timer_indicator_disk_v2 (Autodesk Fusion 360 design; units mm, degrees)
Autodesk Fusion 360 part; units mm, degrees
note: some values were not read from the file. Chosen so that the rebuilt part matches the saved one: that a step has no effect.
sketch "Sketch1" plane through (0, 0, 0) normal (0, 0, 1) x (1, 0, 0)
  circle A0 centre (0, 0) radius 65
  line L0 (2.125, -0.975) -> (2.125, 0.975)
  arc A1 (2.125, 0.975) -> (-2.125, 0.975) centre (0, 0.975) ccw
  line L1 (-2.125, 0.975) -> (-2.125, -0.975)
  arc A2 (-2.125, -0.975) -> (2.125, -0.975) centre (0, -0.975) ccw
  line L2 (0, -0.975) -> (0, 0.975) construction
  line L3 (0, 3.1) -> (0, -3.1) construction
  line L4 (0, 0) -> (65, 0) construction
  line L5 (0, 0) -> (-65, 0) construction
  circle A3 centre (-7.25, 0) radius 1.125
  circle A4 centre (7.25, 0) radius 1.125
  line L6 (-6.125, 0) -> (-2.125, 0) construction
  line L7 (6.125, 0) -> (2.125, 0) construction
  line L8 (12.5, 0) -> (5, -11.8216)
  arc A5 (12.5, 0) -> (-12.5, 0) centre (0, 0) ccw
  line L9 (5, -11.8216) -> (-5, -11.8216)
  line L10 (0, -0.975) -> (0, -65) construction
  line L11 (0, -35.0581) -> (0, -65) construction
  line L12 (-12.5, 0) -> (-5, -11.8216)
  arc A6 (16.4537, -1.2347) -> (-16.5, 0) centre (0, 0) ccw
  line L13 (16.4537, -1.2347) -> (9.6102, -12.0216)
  line L14 (9.6102, -12.0216) -> (-0.3898, -12.0216)
  arc A7 (-0.3898, -12.0216) -> (-0.3898, -21.6037) centre (-0.3898, -16.8127) ccw
  line L15 (-0.3898, -21.6037) -> (0.0565, -21.6037)
  line L16 (0.0565, -21.6037) -> (0.0565, -65)
  line L17 (5, -11.8216) -> (-0.3898, -11.8216)
  arc A8 (-0.3898, -11.8216) -> (-0.1435, -21.7976) centre (-0.3898, -16.8127) ccw
  line L18 (-0.1435, -21.7976) -> (-0.1435, -64.9998)
  line L19 (0.0565, -65) -> (-0.0002, -73)
  arc A9 (-0.0002, -73) -> (3.9997, -73.0283) centre (1.9998, -73.0141) ccw
  line L20 (3.9997, -73.0283) -> (4.0575, -64.8732)
  arc A10 (-16.5, 0) -> (-12.5, 0) centre (-14.5, 0) ccw
  line L21 (0, 12.5) -> (39.231, 12.5) construction
  line L22 (0, -11.8216) -> (39.4618, -11.8216) construction
  dimension "d1" = 130
  dimension "d2" = 4.25
  dimension "d4" = 6.2
  dimension "d5" = 2.25
  dimension "d6" = 2.25
  dimension "d7" = 4
  dimension "d8" = 4
  dimension "d10" = 14
  dimension "d11" = 25
  dimension "d12" = 12.5
  dimension "d13" = 10
  dimension "d14" = 14
  dimension "d15" = 4
  dimension "d16" = 0.2
  dimension "d17" = 0.2
  dimension "d18" = 4
  dimension "d19" = 10
  dimension "d20" = 8
  dimension "d23" = 24.3216
  dimension "d32" = 4
  constraint coincident A0.centre L4.start
  constraint tangent L0 A1
  constraint tangent A1 L1
  constraint parallel L0 L1
  constraint tangent L1 A2
  constraint tangent L0 A2
  constraint vertical L2
  constraint midpoint L2 A0.centre
  constraint midpoint A1 L3.start
  constraint midpoint A2 L3.end
  constraint coincident A0 L4.end
  constraint perpendicular L3 L4
  constraint coincident A0 L5.end
  constraint perpendicular L1 L5
  constraint coincident L5 A3.centre
  constraint coincident L4 A4.centre
  constraint coincident A3 L6.start
  constraint coincident L5 L6.start
  constraint midpoint L1 L6.end
  constraint coincident L4 L7.start
  constraint coincident A4 L7.start
  constraint midpoint L0 L7.end
  constraint coincident L4 L8.start
  constraint coincident L5 A5.end
  constraint horizontal L9
  constraint coincident A2.centre L2.start
  constraint coincident A0 L10.end
  constraint parallel L3 L10
  constraint coincident L11.start L10
  constraint perpendicular L10 L14
  constraint parallel L8 L13
  constraint tangent L14 A7
  constraint tangent A7 L15
  constraint perpendicular L10 L15
  constraint coincident A0 L16.end
  constraint perpendicular L15 L16
  constraint coincident L9 L17.end
  constraint tangent L17 A8
  constraint coincident A0 L18.end
  constraint parallel L16 L18
  constraint coincident A7.centre A8.centre
  constraint tangent L19 A9
  constraint coincident A0 L20.end
  constraint tangent A9 L20
  constraint parallel L19 L20
  constraint tangent A6 A10
  constraint midpoint A5 L21.start
  constraint tangent A5 L21
  constraint horizontal L21
  constraint midpoint L9 L22.start
  constraint perpendicular L10 L22
  measures "d1" diameter of A0
  measures "d2" diameter of A1
  measures "d4" distance of L3.start L3.end
  measures "d5" diameter of A3
  measures "d6" diameter of A4
  measures "d7" distance of L6.start L6.end
  measures "d8" distance of L7.start L7.end
  measures "d10" distance of L8.start L8.end
  measures "d11" distance of L8.start A5.end
  measures "d12" radius of A5
  measures "d13" distance of L8.end L9.end
  measures "d14" distance of A5.end L9.end
  measures "d16" distance of L16 L18
  measures "d17" distance of A7 A8
  measures "d18" distance of L8 L13
  measures "d19" horizontal distance of L13.end A7.centre
  measures "d20" vertical distance of L16.end L19.end
  measures "d23" distance of L21 L22
  measures "d32" distance of L19 L20
extrude "Extrude1" add sketch "Sketch1" along normal blind 0.4 contours A0 L9 L12 A6 L13 L14 A7 L15 L16 A8 L18 A10 | L8 A5 L9 L12 L17 makes body 1
fillet "Fillet1" [no effect]
fillet "Fillet2" radius 3 2 edges at (5, -11.8216, 0.2) (9.6102, -12.0216, 0.2) on bodies 1
fillet "Fillet3" radius 3 2 edges at (12.5, 0, 0.2) (16.4537, -1.2347, 0.2) on bodies 1
extrude "Extrude2" add sketch "Sketch1" along normal blind 0.4 separate body contours A0 L19 A9 L20 makes body 2
combine "Combine1" operation add target body 1 tool bodies 2
